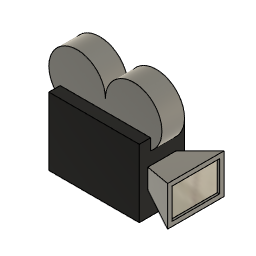
Camera (Autodesk Fusion 360 design; units mm, degrees)
Autodesk Fusion 360 part; units mm, degrees
box "PrimitivaParallelepipedo1" add length 200 width 400 height 300 placed x (0, 1, 0) y (-1, 0, 0) z (0, 0, 1) at (400, 0, 0)
ref_plane "Piano di lavoro1" through (200, 100, 150) normal (0, -1, 0) x (0, 0, 1)
sketch "Schizzo2" plane through (0, 100, 0) normal (0, -1, 0) x (-1, 0, 0)
  line L0 (-400, -300) -> (-400, 0)
  line L1 (-400, 0) -> (0, 0)
  line L2 (0, 0) -> (0, -300)
  line L3 (0, -300) -> (-400, -300)
  line L4 (-325, -350) -> (-75, -350)
  line L5 (-200, -350) -> (-200, -300)
  circle A0 centre (-325, -350) radius 125
  circle A1 centre (-75, -350) radius 125
  line L6 (-325, -225) -> (-75, -225)
  dimension "d6" = 50
  dimension "d7" = 250
  constraint horizontal L4
  constraint midpoint L4 L5.start
  constraint midpoint L3 L5.end
  constraint perpendicular L3 L5
  constraint coincident L4.start A0.centre
  constraint coincident L5.start A0
  constraint coincident L4.end A1.centre
  constraint coincident L5.start A1
  constraint coincident A0 L6.start
  constraint coincident A1 L6.end
  constraint tangent A1 L6
  constraint tangent A0 L6
  measures "d6" distance of L3 L4
  measures "d7" distance of L4.start L4.end
extrude "Estrusione1" add sketch "Schizzo2" along normal mid plane 100 contours L0 L3 A0 | L3 L5 A0 | L2 L3 A1 | L3 L5 A1 picked at (-284.0328, -383.892) picked at (-121.967, -374.8835)
ref_plane "Piano di lavoro2" through (550, 100, 150) normal (1, 0, 0) x (0, 0, -1)
sketch "Schizzo3" plane through (550, 0, 0) normal (1, 0, 0) x (0, 1, 0)
  line L0 (50, 250) -> (50, 300) construction
  line L1 (50, 300) -> (0, 300) construction
  line L2 (0, 300) -> (0, 0) construction
  line L3 (0, 0) -> (200, 0) construction
  line L4 (200, 0) -> (200, 300) construction
  line L5 (200, 300) -> (150, 300) construction
  line L6 (150, 300) -> (150, 250) construction
  line L7 (150, 250) -> (50, 250) construction
  line L8 (0, 300) -> (200, 0) construction
  line L9 (225, 237.5) -> (-25, 237.5)
  line L10 (-25, 237.5) -> (-25, 62.5)
  line L11 (-25, 62.5) -> (225, 62.5)
  line L12 (225, 62.5) -> (225, 237.5)
  line L13 (225, 237.5) -> (-25, 62.5) construction
  line L14 (-25, 237.5) -> (225, 62.5) construction
  point P0 (100, 150)
  dimension "d11" = 250
  dimension "d12" = 175
  constraint coincident L1.end L2.start
  constraint coincident L3.end L4.start
  constraint horizontal L9
  constraint perpendicular L9 L10
  constraint parallel L9 L11
  constraint parallel L10 L12
  constraint coincident L13 P0
  constraint coincident L14 P0
  constraint midpoint L8 P0
  measures "d11" distance of L10.end L11.end
  measures "d12" distance of L9.end L10.end
sketch "Schizzo4" plane through (400, 0, 0) normal (1, 0, 0) x (0, 1, 0)
  line L0 (50, 250) -> (50, 300)
  line L1 (50, 300) -> (0, 300)
  line L2 (0, 300) -> (0, 0)
  line L3 (0, 0) -> (200, 0)
  line L4 (200, 0) -> (200, 300)
  line L5 (200, 300) -> (150, 300)
  line L6 (150, 300) -> (150, 250)
  line L7 (150, 250) -> (50, 250)
  line L8 (200, 300) -> (0, 0) construction
  line L9 (162.5, 193.75) -> (37.5, 193.75)
  line L10 (37.5, 193.75) -> (37.5, 106.25)
  line L11 (37.5, 106.25) -> (162.5, 106.25)
  line L12 (162.5, 106.25) -> (162.5, 193.75)
  line L13 (162.5, 193.75) -> (37.5, 106.25) construction
  line L14 (37.5, 193.75) -> (162.5, 106.25) construction
  point P0 (100, 150)
  dimension "d13" = 125
  dimension "d14" = 87.5
  constraint coincident L4.end L5.start
  constraint coincident L2.end L3.start
  constraint horizontal L9
  constraint perpendicular L9 L10
  constraint parallel L9 L11
  constraint parallel L10 L12
  constraint coincident L13 P0
  constraint coincident L14 P0
  constraint midpoint L8 P0
  measures "d13" distance of L10.end L11.end
  measures "d14" distance of L9.end L10.end
loft "Loft1" add profiles "Schizzo4", "Schizzo3" section 1 contours L9 L10 L11 L12 section 2
sketch "Schizzo5" plane through (550, 0, 0) normal (1, 0, 0) x (0, 1, 0)
  line L0 (225, 62.5) -> (225, 237.5)
  line L1 (225, 237.5) -> (-25, 237.5)
  line L2 (-25, 237.5) -> (-25, 62.5)
  line L3 (-25, 62.5) -> (225, 62.5)
  line L4 (-5, 82.5) -> (205, 82.5)
  line L5 (205, 82.5) -> (205, 217.5)
  line L6 (205, 217.5) -> (-5, 217.5)
  line L7 (-5, 217.5) -> (-5, 82.5)
  dimension "d15" = -20
extrude "Estrusione2" cut sketch "Schizzo5" against normal blind 10 contours L4 L5 L6 L7
component "Component" placed x (1, 0, 0) y (0, 1, 0) z (0, 0, 1) at (0, 0, 0)
equation "d14 = ( 175 / 2 ) * 1 mm"
